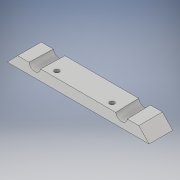
# Autodesk Inventor part: Bar_Mount_Bottom
Saved by Autodesk Inventor 2019 (Build 230136000, 136)
## iProperties
Created: 2019-08-14
Part Number: Bar_Mount_Bottom
Material: Generic
Document SubType Name: Modeling
Designer: steve
Density: 1 g/cm^3
Appearance: Default
Author: steve
Autodesk Inventor part; units mm, degrees
ref_plane "YZ Plane" through (0, 0, 0) normal (1, 0, 0) x (0, 1, 0)
ref_plane "XZ Plane" through (0, 0, 0) normal (0, 1, 0) x (-1, 0, 0)
sketch "Sketch1" plane through (0, 0, 0) normal (0, 0, 1) x (1, 0, 0)
  line L0 (90, -7.3229) -> (-90, -7.3229)
  line L1 (-90, -7.3229) -> (-76.8391, 6.2521)
  line L2 (-76.8391, 6.2521) -> (-61.4824, 6.2521)
  line L3 (76.8391, 6.2521) -> (90, -7.3229)
  line L4 (90, -7.3229) -> (-76.8391, 6.2521) construction
  line L5 (-90, -7.3229) -> (76.8391, 6.2521) construction
  line L6 (-75.8696, 7.2521) -> (77.8086, 7.2521) construction
  arc A0 (-46.7676, 6.2521) -> (-61.4824, 6.2521) centre (-54.125, 7.2521) ccw construction
  arc A1 (47.5169, 3.8663) -> (61.4824, 6.2521) centre (54.125, 7.2521) ccw
  line L7 (46.7676, 6.2521) -> (61.4824, 6.2521) construction
  line L8 (61.4824, 6.2521) -> (76.8391, 6.2521)
  arc A2 (46.7676, 6.2521) -> (47.5169, 3.8663) centre (54.125, 7.2521) ccw
  arc A3 (61.4824, 6.2521) -> (46.7676, 6.2521) centre (54.125, 7.2521) ccw construction
  line L9 (-61.4824, 6.2521) -> (-46.7676, 6.2521) construction
  line L10 (-46.7676, 6.2521) -> (46.7676, 6.2521)
  arc A4 (-47.5169, 3.8663) -> (-46.7676, 6.2521) centre (-54.125, 7.2521) ccw
  arc A5 (-61.1935, 4.9791) -> (-47.5169, 3.8663) centre (-54.125, 7.2521) ccw
  arc A6 (-61.4824, 6.2521) -> (-61.1935, 4.9791) centre (-54.125, 7.2521) ccw
  point P0 (0, 0)
  dimension "d0" = 1
  dimension "d1" = 14.85
  dimension "d2" = 54.125
  dimension "d3" = 108.25
  dimension "d5" = 180
  dimension "d6" = 22.7141
  dimension "d7" = 22.7141
  dimension "d8" = 14.575
  constraints: 22 end point, 15 point on circle, 8 point on line, 7 centre point, 6 horizontal, 5 parallel, 1 equal radius
  measures "d0" distance between parallel lines of L6 L2
  measures "d1" diameter of A0
  measures "d2" horizontal distance of point (0, 0) A0.centre
  measures "d3" distance of A1.centre A0.centre
  measures "d5" distance of L0.start L0.end
  measures "d6" horizontal distance of L1.end A0.centre
  measures "d7" horizontal distance of L3.start A1.centre
  measures "d8" distance from line of A0.centre L0
ref_plane "Work Plane1" through (0, 0, 30) normal (0, 0, 1) x (1, 0, 0)
sketch "Sketch2" plane through (0, 0, 30) normal (0, 0, 1) x (1, 0, 0)
  line L0 (90, -7.3229) -> (-90, -7.3229) projected
  line L1 (-90, -7.3229) -> (-76.8391, 6.2521) projected
  line L2 (76.8391, 6.2521) -> (90, -7.3229) projected
  line L3 (62.3824, 6.2521) -> (76.8391, 6.2521)
  line L4 (-47.6676, 6.2521) -> (47.6676, 6.2521)
  line L5 (-76.8391, 6.2521) -> (-62.3824, 6.2521)
  line L6 (-75.8696, 7.2521) -> (77.8086, 7.2521) construction
  arc A0 (-62.3824, 6.2521) -> (-47.6676, 6.2521) centre (-55.025, 7.2521) ccw
  arc A1 (47.6676, 6.2521) -> (62.3824, 6.2521) centre (55.025, 7.2521) ccw
  point P0 (0, 0)
  dimension "d10" = 7.425
  dimension "d11" = 110.05
  dimension "d12" = 55.025
  constraints: 6 end point, 4 point on circle, 2 centre point, 2 collinear, 2 point on line, 1 equal radius
  measures "d10" radius of A0
  measures "d11" distance of A1.centre A0.centre
  measures "d12" horizontal distance of A0.centre point (0, 0)
loft "Loft1" add profiles "Sketch1", "Sketch2"
sketch "Sketch8" plane through (-90, -7.3229, 0) normal (0, -1, 0) x (1, 0, 0)
  circle A0 centre (125, 22) radius 3
  circle A1 centre (55, 22) radius 3
  point P0 (90, 0)
  dimension "d31" = 35
  dimension "d32" = 35
  dimension "d33" = 22
  dimension "d34" = 22
  dimension "d35" = 6
  constraints: 2 centre point, 1 equal radius
  measures "d31" horizontal distance of point (90, 0) A0.centre
  measures "d32" horizontal distance of point (90, 0) A1.centre
  measures "d33" vertical distance of point (90, 0) A0.centre
  measures "d34" vertical distance of point (90, 0) A1.centre
  measures "d35" diameter of A0
extrude "Extrusion3" cut sketch "Sketch8" against normal through all
sketch "Sketch9" plane through (-90, -7.3229, 0) normal (0, -1, 0) x (1, 0, 0)
  circle A0 centre (125, 22) radius 3 projected
  circle A1 centre (55, 22) radius 3 projected
  line L0 (122.1132, 27) -> (127.8868, 27)
  line L1 (127.8868, 27) -> (130.7735, 22)
  line L2 (130.7735, 22) -> (127.8868, 17)
  line L3 (127.8868, 17) -> (122.1132, 17)
  line L4 (122.1132, 17) -> (119.2265, 22)
  line L5 (119.2265, 22) -> (122.1132, 27)
  line L6 (52.1132, 27) -> (57.8868, 27)
  line L7 (57.8868, 27) -> (60.7735, 22)
  line L8 (60.7735, 22) -> (57.8868, 17)
  line L9 (57.8868, 17) -> (52.1132, 17)
  line L10 (52.1132, 17) -> (49.2265, 22)
  line L11 (49.2265, 22) -> (52.1132, 27)
  point P0 (90, 0)
  dimension "d38" = 10
  constraints: 24 end point, 2 coincident, 2 horizontal, 1 collinear, 26 other
  measures "d38" distance between parallel lines of L0 L3
extrude "Extrusion4" cut sketch "Sketch9" against normal blind 5
equation "\"d2\" = 0.5 * d3"
equation "\"d5\" = topWidth"
equation "\"d7\" = d6"
equation "\"d10\" = 0.5 * d1"
equation "\"d12\" = 0.5 * d11"
equation "\"d32\" = d31"
equation "\"d34\" = d33"
equation "\"topWidth\" = 180"
body "Solid1"
